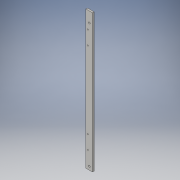
# Autodesk Inventor part: vrRig_v08_enclosure_hingeMount
Saved by Autodesk Inventor 2016 (Build 200138000, 138)
## iProperties
Created: 2018-01-18
Part Number: vrRig_v08_enclosure_hingeMount
Material: Generic
Document SubType Name: Modeling
Designer: harveylab
Density: 1 g/cm^3
Appearance: Default
Author: harveylab
Autodesk Inventor part; units mm, degrees
ref_plane "YZ Plane" through (0, 0, 0) normal (1, 0, 0) x (0, 1, 0)
ref_plane "XZ Plane" through (0, 0, 0) normal (0, 1, 0) x (-1, 0, 0)
ref_plane "XY Plane" through (0, 0, 0) normal (0, 0, 1) x (1, 0, 0)
sketch "Sketch1" plane through (0, 0, 0) normal (0, 0, 1) x (1, 0, 0)
  line L0 (0, 0) -> (24.13, 0)
  line L1 (24.13, 0) -> (24.13, 508)
  line L2 (24.13, 508) -> (0, 508)
  line L3 (0, 508) -> (0, 0)
  line L4 (0, 0) -> (25.4, 0)
  line L5 (25.4, 0) -> (25.4, 25.4)
  line L6 (25.4, 50.8) -> (0, 50.8) construction
  line L7 (0, 25.4) -> (0, 0)
  line L8 (0, 50.8) -> (25.4, 50.8) construction
  line L9 (25.4, 25.4) -> (25.4, 98.425)
  line L10 (25.4, 123.825) -> (0, 123.825) construction
  line L11 (0, 98.425) -> (0, 25.4)
  line L12 (25.4, 98.425) -> (25.4, 87.3125)
  line L13 (25.4, 112.7125) -> (7.3422, 112.7125) construction
  circle A0 centre (7.3422, 112.7125) radius 2.0193
  line L14 (25.4, 87.3125) -> (25.4, 61.9125)
  line L15 (25.4, 87.3125) -> (8.6883, 87.3125) construction
  circle A1 centre (7.3422, 61.9125) radius 2.0193
  line L16 (0, 25.4) -> (0, 50.8)
  line L17 (0, 25.4) -> (12.7, 25.4) construction
  line L18 (0, 0) -> (0, 254)
  line L19 (0, 254) -> (96.9317, 254) construction
  circle A2 centre (7.3422, 395.2875) radius 2.0193
  circle A3 centre (7.3422, 446.0875) radius 2.0193
  circle A4 centre (12.7, 469.9) radius 3.302
  circle A5 centre (12.7, 12.7) radius 3.302
  dimension "d0" = 24.13
  dimension "d1" = 508
  dimension "d2" = 25.4
  dimension "d3" = 73.025
  dimension "d4" = 11.1125
  dimension "d5" = 18.0578
  dimension "d6" = 4.0386
  dimension "d7" = 25.4
  dimension "d8" = 25.4
  dimension "d12" = 254
  dimension "d16" = 6.604
  constraints: 40 end point, 6 centre point, 6 parallel, 6 perpendicular, 4 horizontal, 3 symmetric about line, 1 coincident, 1 midpoint, 1 point on line, 3 other
  measures "d0" distance of L2.end L1.end
  measures "d1" distance of L1.end L0.end
  measures "d2" distance of L5.end L4.end
  measures "d3" distance of L9.start L9.end
  measures "d4" distance of L12.start L12.end
  measures "d5" distance of L13.start L13.end
  measures "d6" diameter of A0
  measures "d7" distance of L14.start L14.end
  measures "d8" distance of L16.start L16.end
  measures "d12" distance of L0.start L18.end
  measures "d16" diameter of A5
extrude "Extrusion2" add sketch "Sketch1" along normal blind 6.35
body "Solid2"
